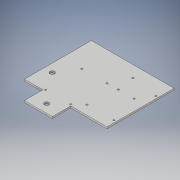
# Autodesk Inventor part: КВ33.044.002 - Дно платы
Saved by Autodesk Inventor 2019 (Build 230136000, 136)
## iProperties
Created: 2019-10-30
Part Number: КВ33.044.002 - Дно платы
Material: Типовые
Document SubType Name: Modeling
Designer: Петров Иван
Density: 1 g/cm^3
Appearance: По умолчанию
Author: Петров Иван
Autodesk Inventor part; units mm, degrees
ref_plane "YZ Plane" through (0, 0, 0) normal (1, 0, 0) x (0, 1, 0)
ref_plane "XZ Plane" through (0, 0, 0) normal (0, 1, 0) x (-1, 0, 0)
ref_plane "XY Plane" through (0, 0, 0) normal (0, 0, 1) x (1, 0, 0)
sketch "Эскиз1" plane through (0, 0, 0) normal (0, 1, 0) x (-1, 0, 0)
  line L0 (-25, 35) -> (25, 35)
  line L1 (25, 35) -> (25, -35)
  line L2 (25, -35) -> (-25, -35)
  line L3 (-25, -35) -> (-25, 35)
  line L4 (-22.5, 32.5) -> (22.5, 32.5)
  line L5 (22.5, 31.5) -> (22.5, -31)
  line L6 (22.5, -32.5) -> (-22.5, -32.5)
  circle A0 centre (22.5, 32.5) radius 1.5
  circle A1 centre (22.5, -32.5) radius 1.5
  circle A2 centre (-22.5, -32.5) radius 1.5
  circle A3 centre (-22.5, 32.5) radius 1.5
  line L7 (-25, 35) -> (-23.7767, 33.2874) construction
  line L8 (-22.5, -31) -> (-22.5, 31)
  line L9 (23.7767, -33.2874) -> (25, -35) construction
  line L10 (25, -30.9585) -> (25, 35)
  line L11 (25, 35) -> (-25, 35)
  line L12 (25, 35) -> (25, -35)
  point P0 (0, 0)
  dimension "d6" = 3
  dimension "d0" = 50
  dimension "d2" = 45
  dimension "d4" = 3
  dimension "d5" = 3
  dimension "d7" = 3
  constraints: 26 end point, 4 coincident, 4 parallel, 4 point on circle, 3 centre point, 3 horizontal, 2 perpendicular, 2 point on line, 1 vertical alignment, 2 other
  measures "d0" distance of L1.end L2.end
  measures "d2" distance of L6.start L6.end
  measures "d4" diameter of A0
  measures "d5" diameter of A1
  measures "d7" diameter of A3
extrude "Выдавливание1" add sketch "Эскиз1" along normal blind 3 contours L0 L1 L2 L3 | L4 A0 L5 A1 L6 A2 L8 A3
sketch "Эскиз2" plane through (0, 3, 0) normal (0, 1, 0) x (1, 0, 0)
  line L0 (-25, -35) -> (25, -35) projected
  line L1 (-25, -35) -> (-28, -35)
  line L2 (-28, -35) -> (-28, 35)
  line L3 (-28, 35) -> (-25, 35)
  line L4 (-25, 35) -> (-25, -35)
  line L5 (-28, -35) -> (-58, -35)
  line L6 (-58, -35) -> (-58, 35)
  line L7 (-58, 35) -> (-28, 35)
  line L8 (-28, 35) -> (-28, -35)
  line L9 (-25, -35) -> (25, -35)
  line L10 (25, -35) -> (25, -38)
  line L11 (25, -38) -> (-25, -38)
  line L12 (-25, -38) -> (-25, -35)
  line L13 (-25, -38) -> (25, -38)
  line L14 (25, -38) -> (25, -68)
  line L15 (25, -68) -> (-25, -68)
  line L16 (-25, -68) -> (-25, -38)
  line L17 (-25, -68) -> (0, -68)
  line L18 (0, -53) -> (-25, -53)
  line L19 (-25, -53) -> (-25, -68)
  circle A0 centre (0, -53) radius 4
  line L20 (-58, 0) -> (-43, 0)
  circle A1 centre (-43, 0) radius 4
  point P0 (0, 0)
  dimension "d18" = 3
  dimension "d19" = 70
  dimension "d20" = 30
  dimension "d21" = 70
  dimension "d22" = 50
  dimension "d23" = 3
  dimension "d24" = 50
  dimension "d25" = 30
  dimension "d26" = 25
  dimension "d27" = 15
  dimension "d28" = 8
  dimension "d29" = 15
  dimension "d30" = 8
  constraints: 40 end point, 9 parallel, 6 horizontal, 4 perpendicular, 2 centre point, 2 coincident, 1 midpoint
  measures "d18" distance of L2.end L3.end
  measures "d19" distance of L1.end L2.end
  measures "d20" distance of L6.end L7.end
  measures "d21" distance of L5.end L6.end
  measures "d22" distance of L10.end L11.end
  measures "d23" distance of L9.end L10.end
  measures "d24" distance of L14.end L15.end
  measures "d25" distance of L13.end L14.end
  measures "d26" distance of L18.end L18.start
  measures "d27" distance of L18.start L17.end
  measures "d28" diameter of A0
  measures "d29" distance of L20.start L20.end
  measures "d30" diameter of A1
extrude "Выдавливание2" add sketch "Эскиз2" against normal blind 3
sketch "Эскиз3" plane through (0, 3, 0) normal (0, 1, 0) x (1, 0, 0)
  line L0 (-58, -35) -> (-25, -35) projected
  line L1 (-25, -35) -> (25, -35)
  line L2 (25, 35) -> (25, -68) projected
  line L3 (25, -35) -> (75, -35)
  line L4 (75, -35) -> (75, 35)
  line L5 (75, 35) -> (25, 35)
  line L6 (25, 35) -> (25, -35)
  point P0 (0, 0)
  dimension "d33" = 50
  constraints: 10 end point, 2 horizontal, 2 parallel, 1 perpendicular, 1 point on line
  measures "d33" distance of L5.end L4.end
extrude "Выдавливание3" add sketch "Эскиз3" against normal blind 3
move faces "Перенос1" translate (0, 0, -50) faces at (30.6667, 2, -35)
move faces "Перенос2" translate (15, 0, 0) faces at (75, 2, -5)
sketch "Эскиз4" plane through (0, 3, 0) normal (0, 1, 0) x (1, 0, 0)
  line L0 (75.6542, 66.4051) -> (73.1142, 68.9451)
  line L1 (73.1142, 68.9451) -> (38.494, 68.9451)
  line L2 (38.494, 68.9451) -> (34.938, 65.3891)
  line L3 (34.938, 65.3891) -> (34.938, -31.1309)
  line L4 (34.938, -31.1309) -> (36.462, -32.6549)
  line L5 (36.462, -32.6549) -> (86.8302, -32.6549)
  line L6 (86.8302, -32.6549) -> (88.3542, -31.1309)
  line L7 (88.3542, -31.1309) -> (88.3542, 64.6416)
  line L8 (88.3542, 64.6416) -> (86.5907, 66.4051)
  line L9 (86.5907, 66.4051) -> (75.6542, 66.4051)
  circle A0 centre (85.8142, 56.6007) radius 1.5621
  circle A1 centre (70.3727, 33.093) radius 1.3153
  circle A2 centre (42.3565, 33.093) radius 1.5621
  circle A3 centre (37.478, 64.0937) radius 1.5621
  circle A4 centre (37.478, -18.5325) radius 1.5621
  circle A5 centre (85.8142, -18.5325) radius 1.5621
  line L10 (38.1266, 59.1154) -> (38.1266, 60.1865)
  line L11 (36.113, 59.1154) -> (38.1266, 59.1154)
  line L12 (36.113, 60.1865) -> (36.113, 59.1154)
  line L13 (38.1266, 60.1865) -> (36.113, 60.1865)
  line L14 (36.113, 54.0354) -> (38.1266, 54.0354)
  line L15 (36.113, 55.1065) -> (36.113, 54.0354)
  line L16 (38.1266, 55.1065) -> (36.113, 55.1065)
  line L17 (38.1266, 54.0354) -> (38.1266, 55.1065)
  line L18 (36.113, 48.9554) -> (38.1266, 48.9554)
  line L19 (36.113, 50.0265) -> (36.113, 48.9554)
  line L20 (38.1266, 50.0265) -> (36.113, 50.0265)
  line L21 (38.1266, 48.9554) -> (38.1266, 50.0265)
  line L22 (36.113, 43.8754) -> (38.1266, 43.8754)
  line L23 (36.113, 44.9465) -> (36.113, 43.8754)
  line L24 (38.1266, 44.9465) -> (36.113, 44.9465)
  line L25 (38.1266, 43.8754) -> (38.1266, 44.9465)
  line L26 (38.3677, 36.0276) -> (38.3677, 37.0695)
  line L27 (36.284, 36.0276) -> (38.3677, 36.0276)
  line L28 (36.284, 37.0695) -> (36.284, 36.0276)
  line L29 (38.3677, 37.0695) -> (36.284, 37.0695)
  line L30 (36.284, 30.9476) -> (38.3677, 30.9476)
  line L31 (36.284, 31.9895) -> (36.284, 30.9476)
  line L32 (38.3677, 31.9895) -> (36.284, 31.9895)
  line L33 (38.3677, 30.9476) -> (38.3677, 31.9895)
  line L34 (36.284, 25.8676) -> (38.3677, 25.8676)
  line L35 (36.284, 26.9095) -> (36.284, 25.8676)
  line L36 (38.3677, 26.9095) -> (36.284, 26.9095)
  line L37 (38.3677, 25.8676) -> (38.3677, 26.9095)
  line L38 (36.284, 20.7876) -> (38.3677, 20.7876)
  line L39 (36.284, 21.8295) -> (36.284, 20.7876)
  line L40 (38.3677, 21.8295) -> (36.284, 21.8295)
  line L41 (38.3677, 20.7876) -> (38.3677, 21.8295)
  line L42 (38.6247, 12.8188) -> (38.6247, 13.9225)
  line L43 (36.5498, 12.8188) -> (38.6247, 12.8188)
  line L44 (36.5498, 13.9225) -> (36.5498, 12.8188)
  line L45 (38.6247, 13.9225) -> (36.5498, 13.9225)
  line L46 (36.5498, 7.7388) -> (38.6247, 7.7388)
  line L47 (36.5498, 8.8425) -> (36.5498, 7.7388)
  line L48 (38.6247, 8.8425) -> (36.5498, 8.8425)
  line L49 (38.6247, 7.7388) -> (38.6247, 8.8425)
  line L50 (36.5498, 2.6588) -> (38.6247, 2.6588)
  line L51 (36.5498, 3.7625) -> (36.5498, 2.6588)
  line L52 (38.6247, 3.7625) -> (36.5498, 3.7625)
  line L53 (38.6247, 2.6588) -> (38.6247, 3.7625)
  circle A6 centre (42.2228, 64.9099) radius 0.5739
  circle A7 centre (42.2228, 62.3699) radius 0.5739
  circle A8 centre (44.7628, 62.3699) radius 0.5739
  circle A9 centre (47.3028, 62.3699) radius 0.5739
  circle A10 centre (49.8428, 62.3699) radius 0.5739
  circle A11 centre (52.3828, 62.3699) radius 0.5739
  circle A12 centre (54.9228, 62.3699) radius 0.5739
  circle A13 centre (57.4628, 62.3699) radius 0.5739
  circle A14 centre (60.0028, 62.3699) radius 0.5739
  circle A15 centre (62.5428, 62.3699) radius 0.5739
  circle A16 centre (65.0828, 62.3699) radius 0.5739
  circle A17 centre (67.6228, 62.3699) radius 0.5739
  circle A18 centre (70.1628, 62.3699) radius 0.5739
  circle A19 centre (72.7028, 62.3699) radius 0.5739
  circle A20 centre (75.2428, 62.3699) radius 0.5739
  circle A21 centre (77.7828, 62.3699) radius 0.5739
  circle A22 centre (80.3228, 62.3699) radius 0.5739
  circle A23 centre (82.8628, 62.3699) radius 0.5739
  circle A24 centre (85.4028, 62.3699) radius 0.5739
  line L54 (85.0097, 49.2384) -> (86.6059, 49.2384)
  line L55 (85.0097, 49.7435) -> (85.0097, 49.2384)
  line L56 (86.6059, 49.7435) -> (85.0097, 49.7435)
  line L57 (86.6059, 49.2384) -> (86.6059, 49.7435)
  line L58 (85.0097, 44.1584) -> (86.6059, 44.1584)
  line L59 (85.0097, 44.6635) -> (85.0097, 44.1584)
  line L60 (86.6059, 44.6635) -> (85.0097, 44.6635)
  line L61 (86.6059, 44.1584) -> (86.6059, 44.6635)
  line L62 (85.0097, 39.0784) -> (86.6059, 39.0784)
  line L63 (85.0097, 39.5835) -> (85.0097, 39.0784)
  line L64 (86.6059, 39.5835) -> (85.0097, 39.5835)
  line L65 (86.6059, 39.0784) -> (86.6059, 39.5835)
  line L66 (86.8517, 30.7677) -> (86.8517, 31.6014)
  line L67 (85.0097, 30.7677) -> (86.8517, 30.7677)
  line L68 (85.0097, 31.6014) -> (85.0097, 30.7677)
  line L69 (86.8517, 31.6014) -> (85.0097, 31.6014)
  line L70 (85.0097, 25.6877) -> (86.8517, 25.6877)
  line L71 (85.0097, 26.5214) -> (85.0097, 25.6877)
  line L72 (86.8517, 26.5214) -> (85.0097, 26.5214)
  line L73 (86.8517, 25.6877) -> (86.8517, 26.5214)
  line L74 (85.0097, 20.6077) -> (86.8517, 20.6077)
  line L75 (85.0097, 21.4414) -> (85.0097, 20.6077)
  line L76 (86.8517, 21.4414) -> (85.0097, 21.4414)
  line L77 (86.8517, 20.6077) -> (86.8517, 21.4414)
  line L78 (85.0097, 15.5277) -> (86.8517, 15.5277)
  line L79 (85.0097, 16.3614) -> (85.0097, 15.5277)
  line L80 (86.8517, 16.3614) -> (85.0097, 16.3614)
  line L81 (86.8517, 15.5277) -> (86.8517, 16.3614)
  line L82 (86.8517, 8.8425) -> (86.8517, 9.8174)
  line L83 (85.0097, 8.8425) -> (86.8517, 8.8425)
  line L84 (85.0097, 9.8174) -> (85.0097, 8.8425)
  line L85 (86.8517, 9.8174) -> (85.0097, 9.8174)
  line L86 (85.0097, 3.7625) -> (86.8517, 3.7625)
  line L87 (85.0097, 4.7374) -> (85.0097, 3.7625)
  line L88 (86.8517, 4.7374) -> (85.0097, 4.7374)
  line L89 (86.8517, 3.7625) -> (86.8517, 4.7374)
  line L90 (85.0097, -1.3175) -> (86.8517, -1.3175)
  line L91 (85.0097, -0.3426) -> (85.0097, -1.3175)
  line L92 (86.8517, -0.3426) -> (85.0097, -0.3426)
  line L93 (86.8517, -1.3175) -> (86.8517, -0.3426)
  line L94 (85.0097, -6.3975) -> (86.8517, -6.3975)
  line L95 (85.0097, -5.4226) -> (85.0097, -6.3975)
  line L96 (86.8517, -5.4226) -> (85.0097, -5.4226)
  line L97 (86.8517, -6.3975) -> (86.8517, -5.4226)
  circle A25 centre (82.6163, -12.0604) radius 0.5437
  circle A26 centre (82.6163, -14.6004) radius 0.5437
  circle A27 centre (80.0763, -12.0604) radius 0.5437
  circle A28 centre (80.0763, -17.1404) radius 0.5437
  circle A29 centre (74.5149, -26.9083) radius 0.4144
  circle A30 centre (71.9749, -26.9083) radius 0.4144
  line L98 (38.981, -25.2619) -> (38.981, -22.6458)
  line L99 (38.2684, -25.2619) -> (38.981, -25.2619)
  line L100 (38.2684, -22.6458) -> (38.2684, -25.2619)
  line L101 (38.981, -22.6458) -> (38.2684, -22.6458)
  line L102 (67.4917, -30.1782) -> (67.4917, -28.3773)
  line L103 (66.6358, -30.1782) -> (67.4917, -30.1782)
  line L104 (66.6358, -28.3773) -> (66.6358, -30.1782)
  line L105 (67.4917, -28.3773) -> (66.6358, -28.3773)
  line L106 (79.6307, -30.406) -> (79.6307, -28.1495)
  line L107 (78.7532, -30.406) -> (79.6307, -30.406)
  line L108 (78.7532, -28.1495) -> (78.7532, -30.406)
  line L109 (79.6307, -28.1495) -> (78.7532, -28.1495)
  line L110 (45.1672, -27.3812) -> (45.1672, -26.9421)
  line L111 (42.3032, -27.3812) -> (45.1672, -27.3812)
  line L112 (42.3032, -26.9421) -> (42.3032, -27.3812)
  line L113 (45.1672, -26.9421) -> (42.3032, -26.9421)
  circle A31 centre (71.9749, -24.3683) radius 0.4144
  line L114 (45.1672, -21.1951) -> (45.1672, -20.5077)
  line L115 (42.3032, -21.1951) -> (45.1672, -21.1951)
  line L116 (42.3032, -20.5077) -> (42.3032, -21.1951)
  line L117 (45.1672, -20.5077) -> (42.3032, -20.5077)
  circle A32 centre (80.0763, -14.6004) radius 0.5437
  circle A33 centre (82.6163, -17.1404) radius 0.5437
  circle A34 centre (74.5149, -24.3683) radius 0.4144
  line L118 (85.0097, -8.9375) -> (86.8517, -8.9375)
  line L119 (85.0097, -7.9626) -> (85.0097, -8.9375)
  line L120 (86.8517, -7.9626) -> (85.0097, -7.9626)
  line L121 (86.8517, -8.9375) -> (86.8517, -7.9626)
  line L122 (85.0097, -3.8575) -> (86.8517, -3.8575)
  line L123 (85.0097, -2.8826) -> (85.0097, -3.8575)
  line L124 (86.8517, -2.8826) -> (85.0097, -2.8826)
  line L125 (86.8517, -3.8575) -> (86.8517, -2.8826)
  line L126 (85.0097, 1.2225) -> (86.8517, 1.2225)
  line L127 (85.0097, 2.1974) -> (85.0097, 1.2225)
  line L128 (86.8517, 2.1974) -> (85.0097, 2.1974)
  line L129 (86.8517, 1.2225) -> (86.8517, 2.1974)
  line L130 (85.0097, 6.3025) -> (86.8517, 6.3025)
  line L131 (85.0097, 7.2774) -> (85.0097, 6.3025)
  line L132 (86.8517, 7.2774) -> (85.0097, 7.2774)
  line L133 (86.8517, 6.3025) -> (86.8517, 7.2774)
  line L134 (85.0097, 12.9877) -> (86.8517, 12.9877)
  line L135 (85.0097, 13.8214) -> (85.0097, 12.9877)
  line L136 (86.8517, 13.8214) -> (85.0097, 13.8214)
  line L137 (86.8517, 12.9877) -> (86.8517, 13.8214)
  line L138 (85.0097, 18.0677) -> (86.8517, 18.0677)
  line L139 (85.0097, 18.9014) -> (85.0097, 18.0677)
  line L140 (86.8517, 18.9014) -> (85.0097, 18.9014)
  line L141 (86.8517, 18.0677) -> (86.8517, 18.9014)
  line L142 (85.0097, 23.1477) -> (86.8517, 23.1477)
  line L143 (85.0097, 23.9814) -> (85.0097, 23.1477)
  line L144 (86.8517, 23.9814) -> (85.0097, 23.9814)
  line L145 (86.8517, 23.1477) -> (86.8517, 23.9814)
  line L146 (85.0097, 28.2277) -> (86.8517, 28.2277)
  line L147 (85.0097, 29.0614) -> (85.0097, 28.2277)
  line L148 (86.8517, 29.0614) -> (85.0097, 29.0614)
  line L149 (86.8517, 28.2277) -> (86.8517, 29.0614)
  line L150 (85.0097, 36.5384) -> (86.6059, 36.5384)
  line L151 (85.0097, 37.0435) -> (85.0097, 36.5384)
  line L152 (86.6059, 37.0435) -> (85.0097, 37.0435)
  line L153 (86.6059, 36.5384) -> (86.6059, 37.0435)
  line L154 (85.0097, 41.6184) -> (86.6059, 41.6184)
  line L155 (85.0097, 42.1235) -> (85.0097, 41.6184)
  line L156 (86.6059, 42.1235) -> (85.0097, 42.1235)
  line L157 (86.6059, 41.6184) -> (86.6059, 42.1235)
  line L158 (85.0097, 46.6984) -> (86.6059, 46.6984)
  line L159 (85.0097, 47.2035) -> (85.0097, 46.6984)
  line L160 (86.6059, 47.2035) -> (85.0097, 47.2035)
  line L161 (86.6059, 46.6984) -> (86.6059, 47.2035)
  line L162 (85.0097, 51.7784) -> (86.6059, 51.7784)
  line L163 (85.0097, 52.2835) -> (85.0097, 51.7784)
  line L164 (86.6059, 52.2835) -> (85.0097, 52.2835)
  line L165 (86.6059, 51.7784) -> (86.6059, 52.2835)
  circle A35 centre (85.4028, 64.9099) radius 0.5739
  circle A36 centre (82.8628, 64.9099) radius 0.5739
  circle A37 centre (80.3228, 64.9099) radius 0.5739
  circle A38 centre (77.7828, 64.9099) radius 0.5739
  circle A39 centre (75.2428, 64.9099) radius 0.5739
  circle A40 centre (72.7028, 64.9099) radius 0.5739
  circle A41 centre (70.1628, 64.9099) radius 0.5739
  circle A42 centre (67.6228, 64.9099) radius 0.5739
  circle A43 centre (65.0828, 64.9099) radius 0.5739
  circle A44 centre (62.5428, 64.9099) radius 0.5739
  circle A45 centre (60.0028, 64.9099) radius 0.5739
  circle A46 centre (57.4628, 64.9099) radius 0.5739
  circle A47 centre (54.9228, 64.9099) radius 0.5739
  circle A48 centre (52.3828, 64.9099) radius 0.5739
  circle A49 centre (49.8428, 64.9099) radius 0.5739
  circle A50 centre (47.3028, 64.9099) radius 0.5739
  circle A51 centre (44.7628, 64.9099) radius 0.5739
  line L166 (86.6059, 54.3184) -> (86.6059, 54.8235)
  line L167 (85.0097, 54.3184) -> (86.6059, 54.3184)
  line L168 (85.0097, 54.8235) -> (85.0097, 54.3184)
  line L169 (86.6059, 54.8235) -> (85.0097, 54.8235)
  line L170 (36.5498, 0.1188) -> (38.6247, 0.1188)
  line L171 (36.5498, 1.2225) -> (36.5498, 0.1188)
  line L172 (38.6247, 1.2225) -> (36.5498, 1.2225)
  line L173 (38.6247, 0.1188) -> (38.6247, 1.2225)
  line L174 (36.5498, 5.1988) -> (38.6247, 5.1988)
  line L175 (36.5498, 6.3025) -> (36.5498, 5.1988)
  line L176 (38.6247, 6.3025) -> (36.5498, 6.3025)
  line L177 (38.6247, 5.1988) -> (38.6247, 6.3025)
  line L178 (36.5498, 10.2788) -> (38.6247, 10.2788)
  line L179 (36.5498, 11.3825) -> (36.5498, 10.2788)
  line L180 (38.6247, 11.3825) -> (36.5498, 11.3825)
  line L181 (38.6247, 10.2788) -> (38.6247, 11.3825)
  line L182 (36.284, 18.2476) -> (38.3677, 18.2476)
  line L183 (36.284, 19.2895) -> (36.284, 18.2476)
  line L184 (38.3677, 19.2895) -> (36.284, 19.2895)
  line L185 (38.3677, 18.2476) -> (38.3677, 19.2895)
  line L186 (36.284, 23.3276) -> (38.3677, 23.3276)
  line L187 (36.284, 24.3695) -> (36.284, 23.3276)
  line L188 (38.3677, 24.3695) -> (36.284, 24.3695)
  line L189 (38.3677, 23.3276) -> (38.3677, 24.3695)
  line L190 (36.284, 28.4076) -> (38.3677, 28.4076)
  line L191 (36.284, 29.4495) -> (36.284, 28.4076)
  line L192 (38.3677, 29.4495) -> (36.284, 29.4495)
  line L193 (38.3677, 28.4076) -> (38.3677, 29.4495)
  line L194 (36.284, 33.4876) -> (38.3677, 33.4876)
  line L195 (36.284, 34.5295) -> (36.284, 33.4876)
  line L196 (38.3677, 34.5295) -> (36.284, 34.5295)
  line L197 (38.3677, 33.4876) -> (38.3677, 34.5295)
  line L198 (36.113, 41.3354) -> (38.1266, 41.3354)
  line L199 (36.113, 42.4065) -> (36.113, 41.3354)
  line L200 (38.1266, 42.4065) -> (36.113, 42.4065)
  line L201 (38.1266, 41.3354) -> (38.1266, 42.4065)
  line L202 (36.113, 46.4154) -> (38.1266, 46.4154)
  line L203 (36.113, 47.4865) -> (36.113, 46.4154)
  line L204 (38.1266, 47.4865) -> (36.113, 47.4865)
  line L205 (38.1266, 46.4154) -> (38.1266, 47.4865)
  line L206 (36.113, 51.4954) -> (38.1266, 51.4954)
  line L207 (36.113, 52.5665) -> (36.113, 51.4954)
  line L208 (38.1266, 52.5665) -> (36.113, 52.5665)
  line L209 (38.1266, 51.4954) -> (38.1266, 52.5665)
  line L210 (36.113, 56.5754) -> (38.1266, 56.5754)
  line L211 (36.113, 57.6465) -> (36.113, 56.5754)
  line L212 (38.1266, 57.6465) -> (36.113, 57.6465)
  line L213 (38.1266, 56.5754) -> (38.1266, 57.6465)
  point P0 (0, 0)
  point P1 (61.6461, 18.1451)
  constraints: 428 end point, 52 centre point
extrude "Выдавливание4" cut sketch "Эскиз4" against normal blind 3 contours A0 | A1 | A2 | A3 | A4 | A5
